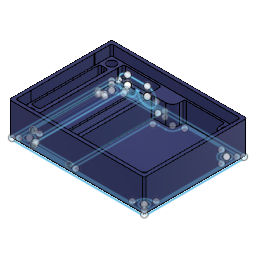
iot-data-logger-enclosure-bottom-base v19 (Autodesk Fusion 360 design; units mm, degrees)
Autodesk Fusion 360 part; units mm, degrees
sketch "Sketch1" plane through (0, 0, 0) normal (0, 1, 0) x (1, 0, 0)
  line L0 (1, 0) -> (78, 0)
  line L1 (79, -0.9985) -> (79, -59.0008)
  line L2 (78, -60) -> (0.9987, -60)
  line L3 (0, -59) -> (0, -1)
  arc A0 (79, -1.0015) -> (78, 0) centre (78, -1) ccw
  arc A1 (78, -60) -> (79, -58.9992) centre (78, -59) ccw
  arc A2 (0, -59) -> (1.0013, -60) centre (1, -59) ccw
  arc A3 (1, 0) -> (0, -1) centre (1, -1) ccw
  circle A4 centre (6, -6) radius 2.5
  line L4 (3, -2) -> (76, -2)
  line L5 (77, -2.9998) -> (77, -57.0015)
  line L6 (76, -58) -> (3, -58)
  line L7 (2, -57) -> (2, -3)
  arc A5 (3, -2) -> (2, -3) centre (3, -3) ccw
  line L8 (3, -2) -> (10, -2)
  line L9 (10, -4) -> (10, -6)
  line L10 (6, -10) -> (4, -10)
  line L11 (2, -10) -> (2, -3)
  arc A6 (2, -11.6976) -> (2, -12.3562) centre (4, -12.0269) ccw
  circle A7 centre (6, -54) radius 2.5
  line L12 (4, -50) -> (6, -50)
  line L13 (10, -54) -> (10, -56)
  arc A8 (2, -48.9994) -> (2, -49.0006) centre (3, -49) ccw
  arc A9 (11, -58) -> (11.0013, -58) centre (11, -57) ccw
  line L14 (69, -56) -> (69, -54)
  line L15 (75, -50) -> (73, -50)
  line L16 (3, -49) -> (3, -10.9995)
  arc A10 (11, -3) -> (10, -4) centre (11, -4) ccw
  arc A11 (4, -10) -> (3, -10.9995) centre (4, -11) ccw
  arc A12 (3, -49) -> (4, -50) centre (4, -49) ccw
  arc A13 (10, -56) -> (11.0013, -57) centre (11, -56) ccw
  arc A14 (2, -57) -> (3, -58) centre (3, -57) ccw
  circle A15 centre (73, -54) radius 2.5
  arc A16 (75, -50) -> (76, -49) centre (75, -49) ccw
  arc A17 (68, -57) -> (69, -56) centre (68, -56) ccw
  arc A18 (73, -50) -> (69, -54) centre (73, -54) ccw
  arc A19 (76, -58) -> (77, -56.9985) centre (76, -57) ccw
  line L17 (69, -6) -> (69, -4)
  line L18 (73, -10) -> (75, -10)
  circle A20 centre (73, -6) radius 2.5
  arc A21 (69, -4) -> (68, -3) centre (68, -4) ccw
  arc A22 (76, -11) -> (75, -10) centre (75, -11) ccw
  line L19 (76, -11) -> (76, -49)
  arc A23 (69, -6) -> (73, -10) centre (73, -6) ccw
  arc A24 (77, -6.003) -> (77, -5.997) centre (73, -6) ccw
  arc A25 (77, -2.9998) -> (76, -2) centre (76, -3) ccw
  line L20 (11, -3) -> (31, -3)
  line L21 (32, -3.9993) -> (32, -56)
  line L22 (10, -56) -> (10, -4)
  arc A26 (32, -4.0007) -> (32, -3.9993) centre (31, -4) ccw
  line L23 (10, -4) -> (10, -4)
  line L24 (10, -4) -> (10, -6)
  line L25 (10, -6) -> (10, -6)
  line L26 (10, -6) -> (10, -4)
  line L27 (32, -4.0007) -> (10, -4.0007)
  line L28 (10, -4.0007) -> (10, -5.5007)
  line L29 (10, -5.5007) -> (32, -5.5007)
  line L30 (32, -5.5007) -> (32, -4.0007)
  line L31 (10, -56) -> (32, -56)
  line L32 (32, -56) -> (32, -54.5)
  line L33 (32, -54.5) -> (10, -54.5)
  line L34 (10, -54.5) -> (10, -56)
  line L35 (11.0013, -57) -> (10.9987, -57)
  arc A27 (31, -57) -> (32, -56) centre (31, -56) ccw
  line L36 (11, -3) -> (31, -3)
  line L37 (46.5, -3) -> (68, -3)
  arc A28 (32, -4.0007) -> (31, -3) centre (31, -4) ccw
  arc A29 (34, -3.9998) -> (34, -4.0002) centre (35, -4) ccw
  arc A30 (34, -55.9992) -> (35, -57) centre (35, -56) ccw
  line L38 (68, -57) -> (35, -57)
  line L39 (31, -57) -> (10.9998, -57)
  line L40 (10, -6.5) -> (9.9686, -6.5)
  line L41 (8, -11) -> (8, -49)
  line L42 (10, -54.5) -> (10, -6.5)
  line L43 (6, -50) -> (7, -50)
  arc A31 (7, -50) -> (8, -49) centre (7, -49) ccw
  line L44 (5.5, -10) -> (7, -10)
  arc A32 (9.9686, -6.5) -> (10, -6) centre (6, -6) ccw
  arc A33 (8, -11) -> (7, -10) centre (7, -11) ccw
  line L45 (37.5, -10) -> (35, -10)
  line L46 (45.5, -6) -> (45.5, -4)
  line L47 (34, -3.9998) -> (34, -4.0002)
  line L48 (34, -10.9998) -> (34, -56.0008)
  line L49 (37.5, -10) -> (41.5, -10)
  arc A34 (41.5, -10) -> (45.5, -6) centre (41.5, -6) ccw
  arc A35 (35, -10) -> (34, -11.0002) centre (35, -11) ccw
  arc A36 (46.5, -3) -> (45.5, -4) centre (46.5, -4) ccw
  dimension "d9" = 73
  dimension "d13" = 1.5
  dimension "d14" = 1.5
  dimension "d51" = 5
  dimension "d52" = 5
  dimension "d53" = 5
  dimension "d54" = 5
  constraint horizontal L0
  constraint vertical L1
  constraint horizontal L2
  constraint vertical L3
  constraint tangent L0 A3
  constraint tangent L2 A1
  constraint tangent L0 A0
  constraint coincident L1.start A0
  constraint coincident L1 A0.start
  constraint coincident L1 A1.end
  constraint coincident A1 L1.end
  constraint coincident L2 A2.end
  constraint coincident A2 L2.end
  constraint horizontal L4
  constraint vertical L5
  constraint horizontal L6
  constraint vertical L7
  constraint tangent L4 A5
  constraint horizontal L8
  constraint vertical L9
  constraint horizontal L10
  constraint vertical L11
  constraint coincident L7 A6.end
  constraint coincident L7 A6.start
  constraint perpendicular L6 L13
  constraint tangent L12 A8
  constraint tangent L13 A9
  constraint coincident L7 A8.start
  constraint coincident L6 A9.end
  constraint tangent L4 A23
  constraint horizontal L36
  constraint vertical L16
  constraint tangent L12 A12
  constraint coincident A9.centre A13
  constraint coincident L7 A8.end
  constraint coincident L6 A9.start
  constraint coincident A13 L39.end
  constraint tangent L6 A14
  constraint tangent L6 A19
  constraint coincident L5 A19.end
  constraint coincident A19 L5.end
  constraint tangent L17 A23
  constraint perpendicular L17 L36
  constraint tangent L18 A23
  constraint tangent A21 L36
  constraint tangent L4 A25
  constraint concentric A20 A23
  constraint coincident L5 A24.start
  constraint concentric A23 A24
  constraint coincident L5 A24.end
  constraint horizontal L20
  constraint vertical L21
  constraint vertical L22
  constraint perpendicular L38 L47
  constraint tangent L20 A26
  constraint tangent A26 L36
  constraint coincident L21 A26.start
  constraint vertical L24
  constraint vertical L26
  constraint horizontal L27
  constraint vertical L28
  constraint horizontal L29
  constraint vertical L30
  constraint horizontal L31
  constraint vertical L32
  constraint horizontal L33
  constraint vertical L34
  constraint coincident L31 A27.centre
  constraint coincident A13 L35.end
  constraint concentric A26 A28
  constraint tangent L20 A28
  constraint collinear L36 L37
  constraint tangent L37 A29
  constraint tangent A30 L38
  constraint coincident A30.start L47
  constraint collinear L38 L39
  constraint coincident A30 L48.end
  constraint horizontal L40
  constraint vertical L41
  constraint vertical L42
  constraint coincident L22 L40.start
  constraint tangent L41 A31
  constraint tangent L44 A33
  constraint perpendicular L45 L46
  constraint tangent L45 A35
  constraint collinear L47 L48
  constraint perpendicular L4 L46
  constraint tangent L49 A34
  constraint coincident L48 A35.end
  constraint coincident A35 L48.start
  measures "d9" distance of A5.centre A25.centre
  measures "d13" distance of A26.start L29.end
  measures "d14" distance of L13.end L33.end
  measures "d51" diameter of A15
  measures "d52" diameter of A7
  measures "d53" diameter of A4
  measures "d54" diameter of A20
sketch "Sketch2" plane through (0, 0, 0) normal (0, 0, 1) x (1, 0, 0)
  line L0 (10, 0, 1) -> (32, 0, 1)
  arc A0 through (21.5, 7.25, 6) (26.75, 2, 6) (32, 7.25, 6)
  arc A1 through (10, 7.25, 6) (15.25, 2, 6) (20.5, 7.25, 6)
  line L1 (20.5, 7.25, 6) -> (21.5, 7.25, 6)
  line L2 (26.75, 7.25, 6) -> (26.75, 7.25, 6)
  line L3 (21.5, 7.25, 6) -> (20.5, 7.25, 6)
  line L4 (15.25, 7.25, 6) -> (15.25, 7.25, 6)
  line L5 (20.5, 7.25, 6) -> (21.5, 7.25, 6)
  line L6 (26.75, 12.4998, 6) -> (15.25, 12.4998, 6)
  arc A2 through (21.5, 7.25, 6) (30.4775, 3.5529, 6) (26.707, 12.4998, 6)
  arc A3 through (15.293, 12.4998, 6) (11.5225, 3.5529, 6) (20.5, 7.25, 6)
extrude "Extrude1" add sketch "Sketch1" along normal blind 2 contours L14 L15 A16 A17 A18 L17 L18 A21 A22 L19 A23 L37 A30 L38 L45 L46 L48 L49 A34 A35 A36 makes body 1
extrude "Extrude2" add sketch "Sketch1" along normal blind 2 separate body contours L10 L12 A8 L16 A11 A12 L41 L43 A31 L44 A33 | A8 L16 A12 picked at (3.3371, -49.0497) makes body 2
extrude "Extrude3" add sketch "Sketch1" along normal blind 19.5 separate body contours L0 L1 L2 L3 A0 A1 A2 A3 makes body 3
extrude "Extrude4" add sketch "Sketch1" along normal blind 13.5 contours A8 L16 A12 | A9 A13 L35 L39 | L4 L5 L6 L7 A5 L8 L11 A14 A19 A24 A25 | A29 picked at (2.3519, -49.1479) picked at (10.9499, -57.6629) bodies 1 2 3
extrude "Extrude5" add sketch "Sketch1" along normal blind 2 contours A9 A13 L31 | A9 A13 L35 L39 | A9 L31 A27 L39 | A26 L27 A28 | A10 L20 A26 L27 L36 picked at (10.9499, -56.3371) bodies 1
extrude "Extrude6" add sketch "Sketch1" along normal blind 7.25 contours L9 L21 L22 L24 L26 L27 L28 L29 L30 | L9 L13 L21 L22 L24 L26 L29 L33 L42 | L13 L21 L22 L31 L32 L33 L34 bodies 1
fillet "Fillet1" radius 1 8 edges at (78.7077, 0, 0.2934) (79, 0, 30.0004) (78.7074, 0, 59.7068) (39.5007, 0, 60) (0.2934, 0, 59.7076) (0, 0, 30) (0.2929, 0, 0.2929) (39.5, 0, 0) on bodies 1
extrude "Extrude13" cut sketch "Sketch2" along normal blind 48 contours A0 A1 L1 L3 L5 L6 A2 A3 in plane through (0, 0, 6) normal (0, 0, 1) bodies 1
extrude "Extrude14" add sketch "Sketch1" along normal blind 8 separate body contours A4 | A7 | A15 | A20 makes body 4 at (75.4969, 5.3333, 54.1246) makes body 5 at (75.4969, 5.3333, 6.1246) makes body 6 at (8.4969, 5.3333, 54.1246) makes body 7 at (8.4969, 5.3333, 6.1246)
combine "Combine4" operation add target body 1 tool bodies 4 6 7 5
named bodies: "bottom-cover"
